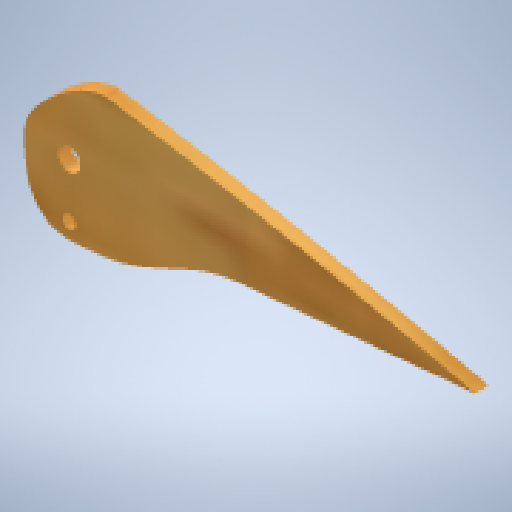
# Autodesk Inventor part: 4P.01.01.02-TW-v1-Basic Structure
Saved by Autodesk Inventor 2025.1 (Build 291241000, 241)
## iProperties
Created: 2024-11-18
Part Number: 4P.01.01.02-TW-v1-Basic Structure
Material: Plywood, Finish
Document SubType Name: Modeling
Designer: thoma
Density: 0.552 g/cm^3
Appearance: Plywood - New
Mass: 2.57337 g
Surface Area: 38.4965 cm^2
Volume: 4.66191 cm^3
Author: thoma
Autodesk Inventor part; units mm, degrees
ref_plane "YZ Plane" through (0, 0, 0) normal (1, 0, 0) x (0, 1, 0)
ref_plane "XZ Plane" through (0, 0, 0) normal (0, 1, 0) x (-1, 0, 0)
ref_plane "XY Plane" through (0, 0, 0) normal (0, 0, 1) x (1, 0, 0)
sketch "Sketch1" plane through (0, 0, 0) normal (0, 0, 1) x (1, 0, 0)
  line L0 (200, 103) -> (200, -97) construction
  line L1 (0, -2198.1975) -> (0, 5744.0191) construction
  line L2 (210, 0) -> (210, -12) construction
  line L3 (210, 0) -> (222, 0) construction
  circle A0 centre (210, -12) radius 1.5
  spline S0 degree 4 poles (218.5257, 15.9738) (214.2153, 16.6356) (204.9526, 10.7069) (199.9456, 4.5262) (200.0001, -0.1196) knots 0 0 0 0 0 0.482971 0.482971 0.482971 0.482971 0.482971
  line L4 (221.1774, 15.5667) -> (215.874, 16.3809) construction
  arc A1 (220.2542, 15.1852) -> (216.6402, 15.74) centre (217.9961, 12.5243) ccw construction
  line L5 (200, 0) -> (200, -15.5) construction
  line L6 (200, -15.5) -> (210, -15.5) construction
  spline S1 degree 2 poles (200, 0) (200, -15.5) (210, -15.5) knots 1 1 1 2 2 2
  line L7 (210, -15.5) -> (228.5627, -15.5) construction
  line L8 (228.5627, -15.5) -> (233.5996, -6.6666) construction
  line L9 (233.5996, -6.6666) -> (247.0398, -5.0019) construction
  spline S2 degree 3 poles (210, -15.5) (228.5627, -15.5) (233.5996, -6.6666) (247.0398, -5.0019) knots 1 1 1 1 2 2 2 2
  line L10 (199.9617, 3.157) -> (200.0386, -3.3962) construction
  arc A2 (200.4959, 2.2656) -> (200.5517, -2.4925) centre (205.6665, -0.0531) ccw construction
  circle A3 centre (210, 0) radius 2.5
  line L11 (-267.3747, 0) -> (404.2133, 0) projected
  spline S3 degree 5 poles (247.0398, -5.0019) (248.7408, -4.851) (252.1086, -4.5511) (256.9966, -4.1115) (263.1536, -3.5406) (270.5088, -2.8843) (276.8391, -2.2398) (282.9867, -1.7375) (287.2724, -1.1764) (292.3303, -0.9034) (294.139, -0.4203) (298.1203, -0.3746) (298.262, -0.0558) (299.6943, -0.05) (299.9984, -0.0244) (300, 0) (300.0016, 0.0244) (299.7036, 0.09) (298.2843, 0.2856) (298.1861, 0.6201) (294.2411, 1.1852) (292.5088, 1.8941) (287.5168, 2.8048) (283.3251, 3.8823) (277.2635, 5.114) (271.0288, 6.4738) (263.7046, 7.9415) (255.8588, 9.4927) (247.2609, 11.1039) (238.144, 12.7436) (230.4968, 14.0478) (224.5814, 15.0163) (220.5538, 15.6564) (218.5257, 15.9738) knots 0.892921 0.892921 0.892921 0.892921 0.892921 0.892921 0.906165 0.919343 0.931928 0.943844 0.955007 0.965319 0.974656 0.982848 0.989595 0.994445 1 1 1 1 1 1.005555 1.010406 1.017155 1.025351 1.034694 1.045016 1.056192 1.068127 1.080735 1.093944 1.107687 1.121902 1.13653 1.151213 1.151213 1.151213 1.151213 1.151213 1.151213
  line L12 (228.403, 14.4279) -> (208.6484, 17.5197) construction
  arc A4 (226.4228, 14.7082) -> (210.6196, 17.1816) centre (49.5564, -1063.5951) ccw construction
  spline S4 degree 5 poles (200, -8.9902) (200.2412, -8.9708) (200.4822, -8.9514) (200.7232, -8.932) (200.9641, -8.9126) (201.2049, -8.8932) knots 1.823971 1.823971 1.823971 1.823971 1.823971 1.823971 1.825664 1.825664 1.825664 1.825664 1.825664 1.825664
  line L13 (199.877, -9.0001) -> (200.123, -8.9803) construction
  arc A5 (199.9016, -8.9981) -> (200.0984, -8.9823) centre (-171.4335, 4609.4167) ccw construction
  point P0 (0, 0)
  point P1 (300, 0)
  point P2 (299.5428, 0.1089)
  point P3 (298.1739, 0.4338)
  point P4 (295.9008, 0.9681)
  point P5 (292.7367, 1.7025)
  point P6 (288.6996, 2.6229)
  point P7 (283.8129, 3.7134)
  point P8 (278.1048, 4.9545)
  point P9 (271.6086, 6.3255)
  point P10 (264.3621, 7.8039)
  point P11 (256.4085, 9.3663)
  point P12 (247.7946, 10.9887)
  point P13 (238.572, 12.6468)
  point P14 (228.7959, 14.3166)
  point P15 (207.8235, 17.5944)
  point P16 (196.755, 19.155)
  point P17 (185.388, 20.6319)
  point P18 (173.7924, 22.0023)
  point P19 (162.0405, 23.2434)
  point P20 (150.2055, 24.3336)
  point P21 (138.3615, 25.2522)
  point P22 (126.5832, 25.98)
  point P23 (114.8976, 26.493)
  point P24 (103.3635, 26.7315)
  point P25 (92.1183, 26.6775)
  point P26 (81.2367, 26.3292)
  point P27 (70.7922, 25.689)
  point P28 (60.8541, 24.7656)
  point P29 (51.489, 23.5734)
  point P30 (42.7587, 22.131)
  point P31 (34.7199, 20.4618)
  point P32 (27.4239, 18.5934)
  point P33 (20.9172, 16.5555)
  point P34 (15.2385, 14.379)
  point P35 (10.422, 12.0954)
  point P36 (6.4944, 9.7347)
  point P37 (3.4767, 7.3239)
  point P38 (1.3836, 4.8867)
  point P39 (0.2238, 2.4411)
  point P40 (0.7011, -2.3487)
  point P41 (2.31, -4.5201)
  point P42 (4.8123, -6.5094)
  point P43 (8.1885, -8.3112)
  point P44 (12.414, -9.9204)
  point P45 (17.4594, -11.3319)
  point P46 (23.2908, -12.5418)
  point P47 (29.871, -13.5477)
  point P48 (37.1583, -14.3505)
  point P49 (45.1092, -14.9526)
  point P50 (53.6766, -15.3609)
  point P51 (62.8101, -15.5853)
  point P52 (72.4581, -15.639)
  point P53 (82.566, -15.5385)
  point P54 (93.0768, -15.3033)
  point P55 (103.9314, -14.9544)
  point P56 (115.0689, -14.514)
  point P57 (126.4866, -13.9956)
  point P58 (138.1008, -13.3755)
  point P59 (149.7945, -12.6672)
  point P60 (161.4972, -11.8896)
  point P61 (173.1378, -11.061)
  point P62 (184.6455, -10.1973)
  point P63 (195.9501, -9.3141)
  point P64 (206.9814, -8.4237)
  point P65 (217.6716, -7.5381)
  point P66 (227.9538, -6.6666)
  point P67 (263.7597, -3.4905)
  point P68 (271.0965, -2.8098)
  point P69 (277.6872, -2.1882)
  point P70 (283.4889, -1.6323)
  point P71 (288.4641, -1.1487)
  point P72 (292.5804, -0.7434)
  point P73 (295.8102, -0.4221)
  point P74 (298.1328, -0.1887)
  point P75 (299.5323, -0.0474)
  point P76 (200.0001, -0.1196)
  dimension "d0" = 200
  dimension "d2" = 200
  dimension "d3" = 12
  dimension "d4" = 90
  dimension "d5" = 10
  dimension "d6" = 3
  dimension "d23" = 5
  dimension "d24" = 12
  constraints: 14 end point, 8 midpoint, 6 centre point, 4 point on circle, 4 point on line, 3 coincident, 2 vertical, 1 collinear, 1 horizontal, 1 perpendicular, 48 other
  measures "d0" distance of L0.start L0.end
  measures "d2" distance between parallel lines of L1 L0
  measures "d3" distance of L2.start L2.end
  measures "d4" angle of L2 L3
  measures "d5" distance between parallel lines of L0 L2
  measures "d6" diameter of A0
  measures "d23" diameter of A3
  measures "d24" distance from line of L11 A0.centre
extrude "Extrusion3" add sketch "Sketch1" along normal blind 3 contours S3 L11 A3 S0 | L11 A3 S3 S2 S1 S0
body "Solid3"
